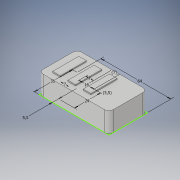
# Autodesk Inventor part: kluc
Saved by Autodesk Inventor 2019 (Build 230136000, 136)
## iProperties
Created: 2020-07-25
Part Number: kluc
Material: Generic
Document SubType Name: Modeling
Designer: lukad
Density: 1 g/cm^3
Appearance: Default
Author: lukad
Autodesk Inventor part; units mm, degrees
ref_plane "YZ Plane" through (0, 0, 0) normal (1, 0, 0) x (0, 1, 0)
ref_plane "XZ Plane" through (0, 0, 0) normal (0, 1, 0) x (-1, 0, 0)
ref_plane "XY Plane" through (0, 0, 0) normal (0, 0, 1) x (1, 0, 0)
sketch "Sketch1" plane through (0, 0, 0) normal (0, 1, 0) x (-1, 0, 0)
  line L0 (34.3512, 32.1074) -> (-29.6488, 32.1074)
  line L1 (-29.6488, 32.1074) -> (-29.6488, -2.8926)
  line L2 (-29.6488, -2.8926) -> (34.3512, -2.8926)
  line L3 (34.3512, -2.8926) -> (34.3512, 32.1074)
  line L4 (27.3512, 26.6074) -> (20.3512, 26.6074)
  line L5 (20.3512, 26.6074) -> (20.3512, 2.6074)
  line L6 (20.3512, 2.6074) -> (27.3512, 2.6074)
  line L7 (27.3512, 2.6074) -> (27.3512, 26.6074)
  line L8 (13.3512, 2.6074) -> (13.3512, 26.6074)
  line L9 (13.3512, 26.6074) -> (6.3512, 26.6074)
  line L10 (6.3512, 2.6074) -> (13.3512, 2.6074)
  line L11 (6.3512, 26.6074) -> (6.3512, 2.6074)
  line L12 (-0.6488, 2.6074) -> (-0.6488, 26.6074)
  line L13 (-0.6488, 26.6074) -> (-7.6488, 26.6074)
  line L14 (-7.6488, 2.6074) -> (-0.6488, 2.6074)
  line L15 (-7.6488, 26.6074) -> (-7.6488, 2.6074)
  point P0 (0, 0)
  dimension "d0" = 35
  dimension "d1" = 64
  dimension "d2" = 7
  dimension "d3" = 7
  dimension "d4" = 24
  dimension "d5" = 5.5
  dimension "d6" = 5.5
  dimension "d9" = 14
  dimension "d14" = 7
  constraints: 32 end point, 4 parallel, 3 horizontal, 2 perpendicular, 16 other
  measures "d0" distance of L2.end L0.start
  measures "d1" distance between parallel lines of L1 L3
  measures "d2" distance between parallel lines of L7 L5
  measures "d3" distance between parallel lines of L3 L7
  measures "d4" distance between parallel lines of L6 L4
  measures "d5" distance between parallel lines of L0 L4
  measures "d6" distance between parallel lines of L2 L6
  measures "d9" distance of L6.end L8.start
  measures "d14" distance between parallel lines of L8 L5
extrude "Extrusion1" add sketch "Sketch1" along normal blind 18
extrude "Extrusion2" add sketch "Sketch1" along normal blind 19 contours L7 L6 L5 L4 | L10 L11 L9 L8 | L14 L15 L13 L12
fillet "Fillet1" radius 4 4 edges at (-34.3512, 9, -2.8926) (-34.3512, 9, 32.1074) (29.6488, 9, -2.8926) (29.6488, 9, 32.1074)
body "Solid1"
